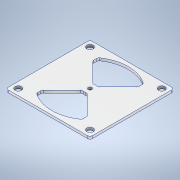
# Autodesk Inventor part: Feeder Bottom Plate
Saved by Autodesk Inventor 2020.3 (Build 243373000, 373)
## iProperties
Created: 2020-07-23
Part Number: Feeder Bottom Plate
Material: Aluminum 6061
Document SubType Name: Modeling
Designer: juanp
Density: 2.7 g/cm^3
Appearance: Aluminum - Flat
Author: juanp
Autodesk Inventor part; units mm, degrees
ref_plane "YZ Plane" through (0, 0, 0) normal (1, 0, 0) x (0, 1, 0)
ref_plane "XZ Plane" through (0, 0, 0) normal (0, 1, 0) x (-1, 0, 0)
ref_plane "XY Plane" through (0, 0, 0) normal (0, 0, 1) x (1, 0, 0)
sketch "Sketch1" plane through (0, 0, 0) normal (0, 1, 0) x (-1, 0, 0)
  arc A0 (20.126, -22.2473) -> (-20.126, -22.2473) centre (0, 0) ccw construction
  circle A1 centre (0, 0) radius 33 construction
  line L0 (33, 33) -> (-33, 33)
  line L1 (-33, 33) -> (-33, -33)
  line L2 (-33, -33) -> (33, -33)
  line L3 (33, -33) -> (33, 33)
  line L4 (33, 33) -> (23.3345, 23.3345) construction
  line L5 (-33, 33) -> (-23.3345, 23.3345) construction
  line L6 (23.3345, 23.3345) -> (-23.3345, -23.3345) construction
  line L7 (23.3345, -23.3345) -> (33, -33) construction
  line L8 (-23.3345, -23.3345) -> (-33, -33) construction
  line L9 (-23.3345, 23.3345) -> (23.3345, -23.3345) construction
  line L10 (0, -33) -> (0, 33) construction
  line L11 (33, 0) -> (-33, 0) construction
  circle A2 centre (0, 0) radius 1.5
  circle A3 centre (0, 0) radius 4.5
  line L12 (4.0607, -1.9393) -> (22.2473, -20.126) construction
  line L13 (1.9393, -4.0607) -> (17.8, -19.9213)
  arc A4 (0, -30) -> (17.8, -24.1487) centre (0, 0) ccw
  line L14 (23.3345, 23.3345) -> (-23.3345, -23.3345) construction
  line L15 (-4.0607, -1.9393) -> (-22.2473, -20.126) construction
  line L16 (-1.9393, -4.0607) -> (-17.8, -19.9213)
  arc A5 (-20.126, -22.2473) -> (-17.8, -24.1487) centre (0, 0) ccw construction
  line L17 (17.8, -24.1487) -> (17.8, -19.9213)
  line L18 (-17.8, -24.1487) -> (-17.8, -19.9213)
  line L19 (17.8, -22.035) -> (-17.8, -22.035) construction
  arc A6 (-17.8, -24.1487) -> (0, -30) centre (0, 0) ccw
  line L20 (-17.8, -19.9213) -> (-20.126, -22.2473) construction
  line L21 (17.8, -19.9213) -> (20.126, -22.2473) construction
  arc A7 (17.8, -24.1487) -> (20.126, -22.2473) centre (0, 0) ccw construction
  line L22 (1.9393, 4.0607) -> (17.8, 19.9213)
  arc A8 (17.8, 24.1487) -> (0, 30) centre (0, 0) ccw
  line L23 (-1.9393, 4.0607) -> (-17.8, 19.9213)
  arc A9 (-17.8, 24.1487) -> (-20.126, 22.2473) centre (0, 0) ccw construction
  line L24 (17.8, 24.1487) -> (17.8, 19.9213)
  line L25 (-17.8, 24.1487) -> (-17.8, 19.9213)
  arc A10 (0, 30) -> (-17.8, 24.1487) centre (0, 0) ccw
  line L26 (-17.8, 19.9213) -> (-20.126, 22.2473) construction
  line L27 (17.8, 19.9213) -> (20.126, 22.2473) construction
  arc A11 (20.126, 22.2473) -> (17.8, 24.1487) centre (0, 0) ccw construction
  circle A12 centre (28.1673, -28.1673) radius 2.55
  circle A13 centre (-28.1673, -28.1673) radius 2.55
  circle A14 centre (-28.1673, 28.1673) radius 2.55
  circle A15 centre (28.1673, 28.1673) radius 2.55
  point P0 (0, -22.035)
  dimension "d22" = 60
  dimension "d24" = 3
  dimension "d25" = 3
  dimension "d26" = 3
  dimension "d27" = 1.5
  dimension "d28" = 3
  dimension "d31" = 35.6
  dimension "d32" = 5.1
  dimension "d33" = 5.1
  dimension "d34" = 5.1
  dimension "d35" = 5.1
  constraints: 56 end point, 26 point on circle, 16 centre point, 13 midpoint, 13 symmetric about line, 8 parallel, 4 coincident, 4 point on line, 4 tangent, 2 horizontal, 1 perpendicular, 1 vertical, 5 other
  measures "d22" diameter of A0
  measures "d24" radial gap between concentric circles of A0 A1
  measures "d25" diameter of A2
  measures "d26" radial gap between concentric circles of A2 A3
  measures "d27" distance between parallel lines of L13 L9
  measures "d28" distance between parallel lines of L13 L12
  measures "d31" distance of L19.start L19.end
  measures "d32" diameter of A12
  measures "d33" diameter of A13
  measures "d34" diameter of A14
  measures "d35" diameter of A15
extrude "Extrusion1" add sketch "Sketch1" along normal blind 2 contours L3 L2 L1 L0 | A3
fillet "Fillet3" radius 2 16 edges at (-17.8, 1, 19.9213) (-1.9393, 1, 4.0607) (1.9393, 1, 4.0607) (-17.8, 1, 24.1487) (17.8, 1, 24.1487) (17.8, 1, 19.9213) (-1.9393, 1, -4.0607) (1.9393, 1, -4.0607) (17.8, 1, -19.9213) (17.8, 1, -24.1487) (-17.8, 1, -19.9213) (-17.8, 1, -24.1487) (-33, 1, 33) (-33, 1, -33) (33, 1, -33) (33, 1, 33)
body "Solid1"
